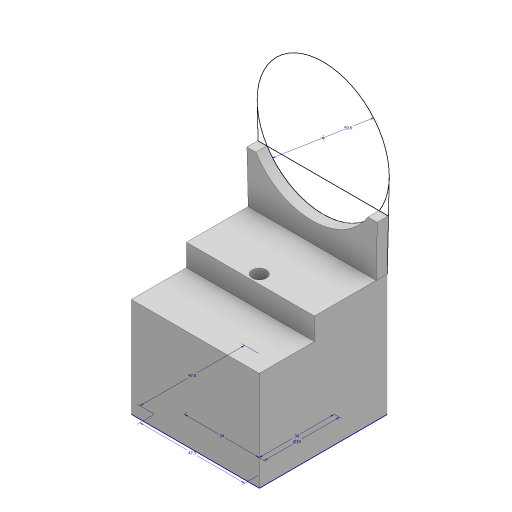
# Autodesk Inventor part: Iris15-XT66P2M_H94mm(axis2base)
Saved by Autodesk Inventor 2023 (Build 270158000, 158)
## iProperties
Created: 2022-05-30
Part Number: Iris15-XT66P2M_H94mm(axis2base)
Material: Generic
Document SubType Name: Modeling
Designer: Nikita
Density: 1 g/cm^3
Appearance: Default
Author: Nikita
Autodesk Inventor part; units mm, degrees
ref_plane "YZ Plane" through (0, 0, 0) normal (1, 0, 0) x (0, 1, 0)
ref_plane "XZ Plane" through (0, 0, 0) normal (0, 1, 0) x (-1, 0, 0)
ref_plane "XY Plane" through (0, 0, 0) normal (0, 0, 1) x (1, 0, 0)
sketch "Sketch1" plane through (0, 0, 0) normal (0, 0, 1) x (1, 0, 0)
  line L0 (29, -29) -> (-29, -29)
  line L1 (-29, -29) -> (-29, 29)
  line L2 (-29, 29) -> (29, 29)
  line L3 (29, 29) -> (29, -29)
  line L4 (29, -29) -> (-29, 29) construction
  line L5 (-29, -29) -> (29, 29) construction
  point P0 (0, 0)
  point P1 (0, 0)
  dimension "d0" = 58
  dimension "d1" = 58
  constraints: 12 end point, 2 midpoint, 2 parallel, 1 coincident, 1 horizontal, 1 perpendicular
  measures "d0" distance of L1.end L2.end
  measures "d1" distance of L0.end L1.end
extrude "Extrusion1" add sketch "Sketch1" along normal blind 55.066
sketch "Sketch2" plane through (0, 0, 55.066) normal (0, 0, 1) x (1, 0, 0)
  line L0 (-29, 29) -> (-29, -29) projected
  line L1 (29, -29) -> (29, 29) projected
  line L2 (-29, -4) -> (29, -4)
  line L3 (29, -4) -> (29, -29)
  line L4 (29, -29) -> (-29, -29)
  line L5 (-29, -29) -> (-29, -4)
  point P0 (0, 0)
  constraints: 8 end point, 2 parallel, 1 horizontal, 1 perpendicular, 1 point on line
extrude "Extrusion2" cut sketch "Sketch2" against normal blind 10
hole "Hole1" at (0, 0, 0) direction (0, 0, 1) diameter 6.5 end through all
sketch "Sketch3" plane through (-29, 29, 0) normal (0, 1, 0) x (1, 0, 0)
  line L0 (0, 0) -> (58, 0) projected
  line L1 (0, 0) -> (0, -55.066) projected
  line L2 (58, -55.066) -> (0, -55.066) projected
  line L3 (58, 0) -> (58, -55.066) projected
  arc A0 (3.5064, -78.162) -> (54.3437, -78.162) centre (28.925, -94.0017) ccw
  line L4 (58, -55.066) -> (58, -45.066) projected
  line L5 (58, -55.066) -> (58.8673, -93.3229)
  line L6 (0, -45.066) -> (0, -55.066) projected
  line L7 (0, -55.066) -> (-1.0173, -94.6805)
  line L8 (58.5236, -78.162) -> (-0.5931, -78.162)
  arc A1 (54.3437, -78.162) -> (3.5064, -78.162) centre (28.925, -94.0017) ccw
  point P0 (29, 0)
  dimension "d13" = 59.9
  constraints: 6 end point, 6 point on circle, 4 point on line, 2 centre point, 1 coincident, 1 horizontal, 1 tangent
  measures "d13" diameter of A0
extrude "Extrusion3" add sketch "Sketch3" against normal blind 5 contours L2 L5 L8 A1 L7
hole "Hole2" at (0, 0, 0) direction (0, 0, 1) diameter 6.756 depth 13 tip angle 118 counterbore diameter 11.113 counterbore depth 11 clearance for "Socket Head Cap Screw" size "1/4" standard "Ansi Unified Screw Threads"
sketch "Sketch4" plane through (0, 0, 0) normal (0, 0, -1) x (-1, 0, 0)
  line L0 (-23.75, 23.75) -> (23.75, 23.75)
  line L1 (23.75, 23.75) -> (23.75, -23.75)
  line L2 (23.75, -23.75) -> (-23.75, -23.75)
  line L3 (-23.75, -23.75) -> (-23.75, 23.75)
  line L4 (-23.75, 23.75) -> (23.75, -23.75) construction
  line L5 (23.75, 23.75) -> (-23.75, -23.75) construction
  line L6 (-14.6492, 0) -> (14.3408, 0)
  point P0 (0, 0)
  point P1 (-17, -17)
  point P2 (17, -17)
  point P3 (-17, 17)
  point P4 (17, 17)
  dimension "d23" = 47.5
  dimension "d24" = 47.5
  dimension "d33" = 34
  dimension "d36" = 34
  dimension "d39" = 34
  constraints: 14 end point, 4 horizontal, 2 midpoint, 2 parallel, 1 perpendicular, 1 point on line, 1 vertical, 3 other
  measures "d23" distance of L1.end L2.end
  measures "d24" distance of L0.end L1.end
  measures "d33" diameter of point (-17, -17) L6
  measures "d36" distance of point (-17, -17) point (17, -17)
  measures "d39" distance of point (-17, -17) point (-17, 17)
hole "Hole3" at (-23.75, -23.75, 0) at (23.75, -23.75, 0) at (-23.75, 23.75, 0) at (23.75, 23.75, 0) direction (0, 0, 1) diameter 2.459 depth 8.8 tip angle 118 thread size "M3x0.5" class "6H" standard "ANSI Metric M Profile"
hole "Hole4" at (17, -17, 0) at (17, 17, 0) at (-17, 17, 0) at (-17, -17, 0) direction (0, 0, 1) diameter 3.242 depth 11.8 tip angle 118 thread size "M4x0.7" class "6H" standard "ANSI Metric M Profile"
body "Solid1"
